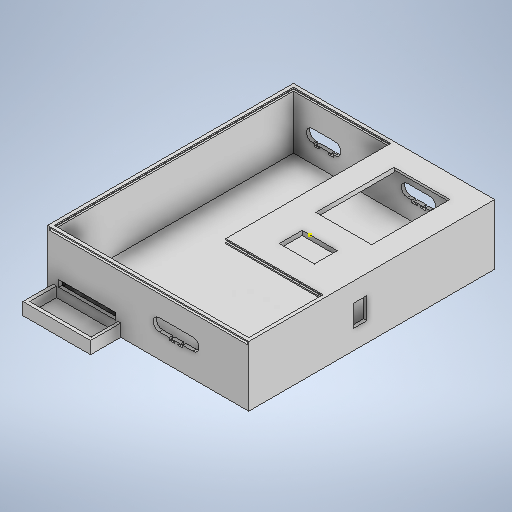
# Autodesk Inventor part: Main Case
Saved by Autodesk Inventor 2025.3 (Build 293356000, 356)
## iProperties
Created: 2026-02-11
Part Number: Main Case
Material: Generic
Document SubType Name: Modeling
Designer: Maulana
Density: 1 g/cm^3
Appearance: Default
Mass: 297.641 g
Surface Area: 2038.3 cm^2
Volume: 297.641 cm^3
Author: Maulana
Autodesk Inventor part; units mm, degrees
sketch "Sketch1" plane through (0, 0, 0) normal (0, 1, 0) x (-1, 0, 0)
  line L0 (-122, 107) -> (122, 107)
  line L1 (122, 107) -> (122, -107)
  line L2 (122, -107) -> (-122, -107)
  line L3 (-122, -107) -> (-122, 107)
  line L4 (-122, 107) -> (122, -107) construction
  line L5 (122, 107) -> (-122, -107) construction
  line L6 (-125, 110) -> (125, 110)
  line L7 (125, 110) -> (125, -110)
  line L8 (125, -110) -> (-125, -110)
  line L9 (-125, -110) -> (-125, 110)
  line L10 (-125, 110) -> (125, -110) construction
  line L11 (125, 110) -> (-125, -110) construction
  line L12 (122, 107) -> (-52, 107)
  line L13 (-52, 107) -> (-52, -107)
  line L14 (125, 110) -> (-55, 110)
  line L15 (-55, 110) -> (-55, -110)
  point P0 (0, 0)
  dimension "d0" = 244
  dimension "d1" = 214
  dimension "d2" = 250
  dimension "d3" = 220
  dimension "d111" = 174
  dimension "d112" = 180
  constraints: 32 end point, 4 midpoint, 4 parallel, 4 perpendicular, 4 point on line, 2 horizontal
  measures "d0" distance of L1.end L2.end
  measures "d1" distance of L0.end L1.end
  measures "d2" distance of L7.end L8.end
  measures "d3" distance of L6.end L7.end
  measures "d111" distance of L0.end L12.end
  measures "d112" distance of L6.end L14.end
extrude "Extrusion1" add sketch "Sketch1" along normal blind 54 contours L0 L15 L6 L7 L8 L2 L1 | L13 L2 L15 L0
sketch "Sketch2" plane through (0, 0, 0) normal (0, -1, 0) x (1, 0, 0)
  line L0 (123.5, 110) -> (-123.5, 110)
  line L1 (-123.5, 110) -> (-123.5, -110)
  line L2 (-123.5, -110) -> (123.5, -110)
  line L3 (123.5, -110) -> (123.5, 110)
  line L4 (123.5, 110) -> (-123.5, -110) construction
  line L5 (-123.5, 110) -> (123.5, -110) construction
  line L6 (55, 110) -> (55, -110) projected
  line L7 (55, 110) -> (55, -110)
  point P0 (0, 0)
  dimension "d6" = 247
  dimension "d7" = 220
  constraints: 14 end point, 2 midpoint, 2 parallel, 2 perpendicular, 1 horizontal
  measures "d6" distance of L2.end L1.end
  measures "d7" distance of L1.end L0.end
extrude "Extrusion2" add sketch "Sketch2" against normal blind 3 contours L6 L2 L1 L0
sketch "Sketch3" plane through (-125, 0, 110) normal (0, 0, 1) x (1, 0, 0)
  line L0 (0, 0) -> (0, 54) projected
  line L1 (0, 27) -> (100, 27)
  circle A0 centre (100, 27) radius 8
  circle A1 centre (100, 27) radius 5.5
  line L2 (100, 35) -> (115, 35)
  line L3 (115, 35) -> (115, 19)
  line L4 (115, 19) -> (100, 19)
  line L5 (100, 19) -> (100, 35)
  line L6 (100, 32.5) -> (115, 32.5)
  line L7 (115, 32.5) -> (115, 21.5)
  line L8 (115, 21.5) -> (100, 21.5)
  line L9 (100, 21.5) -> (100, 32.5)
  line L10 (100, 32.5) -> (109, 32.5)
  line L11 (109, 32.5) -> (109, 34.5)
  line L12 (109, 34.5) -> (113.5, 34.5)
  line L13 (113.5, 34.5) -> (113.5, 33.5)
  line L14 (113.5, 33.5) -> (111, 33.5)
  line L15 (111, 33.5) -> (111, 32.5)
  line L16 (100, 27) -> (115, 27)
  line L17 (109, 21.5) -> (109, 19.5)
  line L18 (109, 19.5) -> (113.5, 19.5)
  line L19 (113.5, 19.5) -> (113.5, 20.5)
  line L20 (113.5, 20.5) -> (111, 20.5)
  line L21 (111, 20.5) -> (111, 21.5)
  point P0 (125, 0)
  dimension "d10" = 100
  dimension "d11" = 16
  dimension "d12" = 11
  dimension "d13" = 15
  dimension "d14" = 9
  dimension "d15" = 2
  dimension "d16" = 4.5
  dimension "d17" = 2.5
  constraints: 42 end point, 6 symmetric about line, 5 parallel, 5 perpendicular, 4 point on circle, 4 point on line, 3 horizontal, 2 centre point, 2 coincident, 2 midpoint, 1 vertical
  measures "d10" distance of L1.start L1.end
  measures "d11" diameter of A0
  measures "d12" diameter of A1
  measures "d13" distance of L3.end L4.end
  measures "d14" distance of L6.start L10.end
  measures "d15" distance of L10.end L11.end
  measures "d16" distance of L11.end L12.end
  measures "d17" distance of L13.end L14.end
extrude "Extrusion3" cut sketch "Sketch3" against normal blind 38 contours A1 L5 L1 | L1 L5 A1 | L16 A1 L5 | L5 A1 L16 | L6 A0 L16 A1 | A1 L16 A0 L8 | L6 L3 L16 A0 | A0 L16 L3 L8 | L8 L21 L20 L19 L18 L17
ref_plane "Work Plane2" through (-10, 21.5, 110) normal (-1, 0, 0) x (0, 0, 1)
mirror "Mirror1" about plane through (-10, 21.5, 110) normal (-1, 0, 0) of "Extrusion3"
sketch "Sketch5" plane through (125, 0, -110) normal (0, 0, -1) x (-1, 0, 0)
  line L0 (250, 6) -> (250, 25)
  line L1 (250, 25) -> (230, 25)
  circle A0 centre (230, 25) radius 8
  circle A1 centre (230, 25) radius 5.5
  line L2 (230, 33) -> (220, 33)
  line L3 (220, 33) -> (220, 17)
  line L4 (220, 17) -> (230, 17)
  line L5 (230, 17) -> (230, 33)
  line L6 (230, 30.5) -> (220, 30.5)
  line L7 (220, 30.5) -> (220, 19.5)
  line L8 (220, 19.5) -> (230, 19.5)
  line L9 (230, 19.5) -> (230, 30.5)
  line L10 (230, 30.5) -> (228.5, 30.5)
  line L11 (228.5, 30.5) -> (228.5, 32.5)
  line L12 (228.5, 32.5) -> (224, 32.5)
  line L13 (224, 32.5) -> (224, 31.5)
  line L14 (224, 31.5) -> (226.5, 31.5)
  line L15 (226.5, 31.5) -> (226.5, 30.5)
  line L16 (230, 25) -> (230, 0)
  line L17 (70, 0) -> (250, 0) projected
  line L18 (250, 0) -> (230, 0)
  line L19 (250, 0) -> (230, 0)
  line L20 (228.5, 19.5) -> (228.5, 17.5)
  line L21 (228.5, 17.5) -> (224, 17.5)
  line L22 (224, 17.5) -> (224, 18.5)
  line L23 (224, 18.5) -> (226.5, 18.5)
  line L24 (226.5, 18.5) -> (226.5, 19.5)
  point P0 (125, 0)
  point P1 (121.8464, -1.1281)
  point P2 (220.8464, 22.8719)
  point P3 (228.3464, 12.8719)
  point P4 (227.2161, 32.5)
  point P5 (225.3363, 31.5)
  point P6 (0, 0)
  point P7 (1.5, 0)
  dimension "d36" = 20
  dimension "d37" = 16
  dimension "d38" = 11
  dimension "d39" = 10
  dimension "d40" = 1.5
  dimension "d41" = 2
  dimension "d42" = 4.5
  dimension "d43" = 2.5
  dimension "d44" = 1
  dimension "d45" = 1
  dimension "d63" = 25
  dimension "d103" = 19
  dimension "d106" = 20
  constraints: 48 end point, 8 perpendicular, 6 point on line, 6 symmetric about line, 4 parallel, 4 point on circle, 3 horizontal, 2 centre point, 2 coincident, 2 collinear
  measures "d36" distance of L0.end L1.end
  measures "d37" diameter of A0
  measures "d38" diameter of A1
  measures "d39" distance of L4.end L3.end
  measures "d40" distance of L6.start L10.end
  measures "d41" distance of L10.end L11.end
  measures "d42" distance of L11.end L12.end
  measures "d43" distance of L13.end L14.end
  measures "d44" distance of L14.end L15.end
  measures "d45" distance of L12.end L13.end
  measures "d63" distance of L16.start L16.end
  measures "d103" distance of L0.start L0.end
  measures "d106" distance of L17.end L16.end
extrude "Extrusion5" cut sketch "Sketch5" against normal blind 10 contours A1 L5 L1 | L1 L5 A1 | L5 A1 | A1 L8 A0 L6 | L21 L22 L23 A0 | A0 L23 L24 L8 L20 L21 | L6 A0 L8 L3
ref_plane "Work Plane4" through (-95, 19.5, -110) normal (-1, 0, 0) x (0, 0, 1)
mirror "Mirror3" about plane through (-95, 19.5, -110) normal (-1, 0, 0) of "Extrusion5"
sketch "Sketch6" plane through (125, 0, -110) normal (0, 0, -1) x (-1, 0, 0)
  circle A0 centre (125, 25) radius 8
  circle A1 centre (125, 25) radius 5.5
  line L0 (125, 33) -> (135, 33)
  line L1 (135, 33) -> (135, 17)
  line L2 (135, 17) -> (125, 17)
  line L3 (125, 30.5) -> (135, 30.5)
  line L4 (135, 19.5) -> (125, 19.5)
  line L5 (125, 30.5) -> (129, 30.5)
  line L6 (129, 30.5) -> (129, 32.5)
  line L7 (129, 32.5) -> (133.5, 32.5)
  line L8 (133.5, 25) -> (133.5, 24.983)
  line L9 (133.5, 31.5) -> (131, 31.5)
  line L10 (131, 31.5) -> (131, 30.5)
  line L11 (116.2614, 18.9998) -> (135.2614, 18.9998) construction
  line L12 (133.5, 32.5) -> (133.5, 31.5)
  line L13 (250, 0) -> (250, 54) projected
  line L14 (250, 0) -> (125, 0)
  line L15 (70, 0) -> (250, 0) projected
  line L16 (125, 25) -> (125, 0)
  line L17 (125, 33) -> (125, 25)
  line L18 (125, 30.5) -> (125, 33)
  line L19 (131, 30.5) -> (131, 31.5)
  line L20 (135, 33) -> (135, 17)
  line L21 (125, 17) -> (135, 17)
  line L22 (125, 25) -> (135, 25)
  line L23 (129, 19.5) -> (129, 17.5)
  line L24 (129, 17.5) -> (133.5, 17.5)
  line L25 (133.5, 18.5) -> (131, 18.5)
  line L26 (131, 18.5) -> (131, 19.5)
  line L27 (133.5, 17.5) -> (133.5, 18.5)
  point P0 (125, 0)
  point P1 (219.2081, 3.6104)
  point P2 (112.7081, 17.6104)
  point P3 (127.7081, 27.6104)
  point P4 (0, 0)
  point P5 (1.5, 0)
  dimension "d50" = 16
  dimension "d51" = 11
  dimension "d54" = 2
  dimension "d55" = 4.5
  dimension "d56" = 2.5
  dimension "d57" = 1.5
  dimension "d104" = 25
  dimension "d105" = 125
  constraints: 52 end point, 6 perpendicular, 6 symmetric about line, 5 point on line, 4 collinear, 4 horizontal, 3 parallel, 2 point on circle, 2 vertical, 1 centre point, 1 coincident, 1 midpoint, 1 vertical alignment, 2 other
  measures "d51" diameter of A1
  measures "d54" distance of L5.end L6.end
  measures "d55" distance of L6.end L7.end
  measures "d56" distance of L9.start L9.end
  measures "d57" distance between parallel lines of L1 L8
  measures "d104" distance of L16.start L14.end
  measures "d105" distance of L13.start L14.end
extrude "Extrusion6" cut sketch "Sketch6" against normal blind 10 contours L3 A0 L22 A1 | L17 L16 A1 | A1 L22 L17 | L23 L4 A0 | A0 L4 L26 L25 L27 L24 L23 | L16 L22 A1 | A1 L22 A0 L4 | L3 L1 L22 A0 | A0 L22 L1 L4
ref_plane "Work Plane5" through (-10, 19.5, -110) normal (1, 0, 0) x (0, 0, -1)
mirror "Mirror4" about plane through (-10, 19.5, -110) normal (1, 0, 0) of "Extrusion6"
sketch "Sketch7" plane through (122, 50, 107) normal (0, 0, -1) x (-1, 0, 0)
  line L0 (70, -47) -> (244, -47) projected
  line L1 (75.0855, -47) -> (75.0855, -50)
  line L2 (75.0855, -50) -> (75.0855, -47)
  line L3 (0, -47) -> (184, -47)
  line L4 (184, -47) -> (184, -39)
  line L5 (184, -39) -> (239, -39)
  line L6 (239, -39) -> (239, -47)
  line L7 (184, -39) -> (194, -39)
  line L8 (239, -39) -> (229, -39)
  line L9 (194, -34.8824) -> (194, -33)
  line L10 (194, -33) -> (229, -33)
  line L11 (229, -33) -> (229, -34.8824)
  line L12 (244, -47) -> (244, 4) projected
  line L13 (184, -47) -> (211.5, -47)
  line L14 (211.5, -47) -> (211.5, -39)
  line L15 (237, -39) -> (237, -33)
  line L16 (237, -33) -> (186, -33)
  line L17 (186, -33) -> (186, -39)
  line L18 (186, -45) -> (237, -33) construction
  line L19 (237, -45) -> (186, -33) construction
  line L20 (186, -39) -> (237, -39)
  point P0 (122, -50)
  point P1 (244, 4)
  point P2 (239, -43)
  point P3 (2, -35)
  point P4 (245, -35)
  point P5 (247, -38)
  point P6 (186, -39)
  point P7 (237, -39)
  dimension "d65" = 8
  dimension "d66" = 55
  dimension "d67" = 10
  dimension "d68" = 10
  dimension "d69" = 6
  dimension "d89" = 5
  dimension "d90" = 51
  constraints: 38 end point, 7 point on line, 4 midpoint, 3 perpendicular, 3 vertical, 2 collinear, 1 horizontal, 1 parallel, 6 other
  measures "d65" distance of L3.end L4.end
  measures "d66" distance of L4.end L5.end
  measures "d67" distance of L4.end L7.end
  measures "d68" distance of L5.end L8.end
  measures "d69" distance of L7.end L9.end
  measures "d90" distance of L18.start L19.start
extrude "Extrusion7" cut sketch "Sketch7" against normal blind 10 contours L5 L17 L16 L10 L15
sketch "Sketch17" plane through (-125, 0, 110) normal (0, 0, 1) x (1, 0, 0)
  line L0 (10, 11) -> (61, 11) projected
  line L1 (35.5, 11) -> (35.5, 0)
  line L2 (177, 3) -> (3, 3) projected
  line L3 (35.5, -2) -> (63, -2)
  line L4 (63, -2) -> (63, 2)
  line L5 (63, 2) -> (8, 2)
  line L6 (8, 2) -> (8, -2)
  line L7 (8, -2) -> (63, 2) construction
  line L8 (63, -2) -> (8, 2) construction
  line L9 (180, 0) -> (0, 0) projected
  line L10 (8, 0) -> (63, 0)
  point P0 (125, 0)
  point P1 (247, 3)
  point P2 (250, 0)
  point P3 (248.5, 0)
  dimension "d91" = 55
  dimension "d92" = 4
  constraints: 16 end point, 5 midpoint, 3 point on line, 2 parallel, 2 perpendicular, 1 horizontal
  measures "d91" distance of L6.end L3.end
  measures "d92" distance of L3.end L4.end
extrude "Extrusion11" add sketch "Sketch17" along normal blind 24
sketch "Sketch18" plane through (-117, 2, 110) normal (0, 1, 0) x (1, 0, 0)
  line L0 (0, 0) -> (0, -24) projected
  line L1 (0, 0) -> (55, 0)
  line L2 (55, 0) -> (55, -24)
  line L3 (55, -24) -> (0, -24)
  line L4 (0, -24) -> (0, 0)
  line L5 (0, 0) -> (-3, 0)
  line L6 (55, 0) -> (58, 0)
  line L7 (-3, 0) -> (57.4885, 0)
  line L8 (57.4885, 0) -> (57.4885, -27)
  line L9 (57.4885, -27) -> (-3, -27)
  line L10 (-3, -27) -> (-3, 0)
  point P0 (117, 110)
  point P1 (57.4885, 0)
  dimension "d95" = 3
  dimension "d96" = 3
  dimension "d97" = 27
  constraints: 20 end point, 4 horizontal, 4 parallel, 2 perpendicular
  measures "d95" distance of L0.start L5.end
  measures "d96" distance of L1.end L6.end
  measures "d97" distance of L7.end L8.end
extrude "Extrusion12" add sketch "Sketch18" along normal blind 9 and the other way blind 2 contours L0 L3 L2 L6 L8 L9 L10 L5
sketch "Sketch20" plane through (0, 54, 0) normal (0, 1, 0) x (1, 0, 0)
  point P0 (0, 0)
sketch "Sketch21" plane through (0, 54, 0) normal (0, 1, 0) x (1, 0, 0)
  line L0 (55, 110) -> (-125, 110) projected
  line L1 (55, 110) -> (-35, 110)
  line L2 (-35, 110) -> (-35, -40.5)
  line L3 (-35, -40.5) -> (55, -40.5)
  line L4 (55, -40.5) -> (55, 110)
  point P0 (0, 0)
  dimension "d113" = 90
  dimension "d114" = 150.5
  constraints: 8 end point, 2 parallel, 1 horizontal, 1 perpendicular
  measures "d113" distance of L3.end L2.end
  measures "d114" distance of L2.end L1.end
extrude "Extrusion14" add sketch "Sketch21" against normal blind 4
sketch "Sketch22" plane through (0, 54, 0) normal (0, 1, 0) x (1, 0, 0)
  line L0 (55, 110) -> (-125, 110) projected
  line L1 (-35, 110) -> (10, 110)
  line L2 (10, 110) -> (10, -40.5)
  line L3 (52, -40.5) -> (-35, -40.5) projected
  line L4 (10, 110) -> (10, 90)
  line L5 (-35, -40.5) -> (-35, 107) projected
  line L6 (-35, 90) -> (-15, 90)
  line L7 (-35, 90) -> (-15, 90) construction
  line L8 (55, -110) -> (55, 110) projected
  line L9 (55, 90) -> (35, 90)
  line L10 (55, 90) -> (75, 90) construction
  line L11 (-15, 90) -> (35, 90)
  line L12 (35, 90) -> (35, 20)
  line L13 (35, 20) -> (-15, 20)
  line L14 (-15, 20) -> (-15, 90)
  point P0 (0, 0)
  dimension "d117" = 45
  dimension "d118" = 20
  dimension "d119" = 20
  dimension "d120" = 0
  dimension "d121" = 20
  dimension "d122" = 180
  dimension "d123" = 70
  constraints: 22 end point, 5 point on line, 4 perpendicular, 3 horizontal, 2 collinear, 2 parallel, 1 midpoint
  measures "d117" distance of L1.start L1.end
  measures "d118" distance of L1.end L4.end
  measures "d119" distance of L6.start L6.end
  measures "d120" distance between parallel lines of L6 L7
  measures "d121" distance of L9.start L9.end
  measures "d122" angle of L9 L10
  measures "d123" distance of L11.end L12.end
extrude "Extrusion15" cut sketch "Sketch22" against normal blind 4 contours L11 L12 L13 L2 | L2 L13 L14 L11
sketch "Sketch23" plane through (0, 54, 0) normal (0, 1, 0) x (1, 0, 0)
  line L0 (52, -40.5) -> (-35, -40.5) projected
  line L1 (8.5, -40.5) -> (8.5, 20)
  line L2 (-15, 20) -> (35, 20) projected
  line L3 (-35, -40.5) -> (-35, 107) projected
  line L4 (-35, -10.25) -> (55, -10.25)
  line L5 (-35, -10.25) -> (55, -10.25) construction
  line L6 (24.25, -20.5) -> (-7.25, -20.5)
  line L7 (-7.25, -20.5) -> (-7.25, 0)
  line L8 (-7.25, 0) -> (24.25, 0)
  line L9 (24.25, 0) -> (24.25, -20.5)
  line L10 (24.25, -20.5) -> (-7.25, 0) construction
  line L11 (-7.25, -20.5) -> (24.25, 0) construction
  point P0 (0, 0)
  point P1 (8.5, -10.25)
  dimension "d126" = 90
  dimension "d127" = 0
  dimension "d128" = 31.5
  constraints: 18 end point, 4 midpoint, 3 point on line, 2 horizontal, 2 parallel, 2 perpendicular, 1 collinear, 1 vertical
  measures "d126" distance of L4.start L4.end
  measures "d127" distance between parallel lines of L4 L5
  measures "d128" distance of L7.end L8.end
extrude "Extrusion16" cut sketch "Sketch23" against normal blind 4 contours L6 L7 L4 L1 | L1 L4 L9 L6 | L4 L7 L8 L1 | L1 L8 L9 L4
sketch "Sketch24" plane through (55, 0, 110) normal (1, 0, 0) x (0, 0, -1)
  line L0 (99.75, 54.0966) -> (99.75, 0)
  line L1 (217, 3) -> (3, 3) projected
  line L2 (0, 0) -> (0, 54) projected
  line L3 (0, 27) -> (220, 27)
  line L4 (220, 0) -> (220, 54) projected
  line L5 (93.75, 17.25) -> (105.75, 17.25)
  line L6 (105.75, 17.25) -> (105.75, 36.75)
  line L7 (105.75, 36.75) -> (93.75, 36.75)
  line L8 (93.75, 36.75) -> (93.75, 17.25)
  line L9 (93.75, 17.25) -> (105.75, 36.75) construction
  line L10 (105.75, 17.25) -> (93.75, 36.75) construction
  point P0 (110, 0)
  point P1 (99.75, 27)
  dimension "d131" = 12
  dimension "d132" = 19.5
  constraints: 16 end point, 4 midpoint, 2 parallel, 2 perpendicular, 2 point on line, 1 horizontal
  measures "d131" distance of L7.end L6.end
  measures "d132" distance of L6.end L5.end
extrude "Extrusion17" cut sketch "Sketch24" against normal blind 4
sketch "Sketch27" plane through (-35, 54, -107) normal (-1, 0, 0) x (0, 0, 1)
  line L0 (17, 0) -> (17, -4) projected
  line L1 (17, -4) -> (7, -4)
  line L2 (147.5, -4) -> (0, -4) projected
  line L3 (7, -4) -> (17, -4)
  line L4 (17, -4) -> (17, -2)
  line L5 (17, -2) -> (7, -2)
  line L6 (7, -2) -> (7, -4)
  point P0 (107, -54)
  dimension "d135" = 10
  constraints: 10 end point, 2 parallel, 1 horizontal, 1 midpoint, 1 perpendicular, 1 point on line
  measures "d135" distance of L0.end L1.end
extrude "Extrusion18" cut sketch "Sketch27" against normal blind 70
sketch "Sketch29" plane through (-125, 54, 110) normal (0, 0, 1) x (1, 0, 0)
  line L0 (3, -51) -> (3, 0) projected
  line L1 (3, 0) -> (3, -1)
  line L2 (3, -1) -> (1.5, -1)
  line L3 (1.5, -1) -> (1.5, -3)
  line L4 (1.5, -3) -> (3, -3)
  line L5 (1.5, -1) -> (178.5, -1)
  line L6 (178.5, -1) -> (178.5, -3)
  line L7 (178.5, -3) -> (1.5, -3)
  line L8 (1.5, -3) -> (1.5, -1)
  line L9 (90, -4) -> (90, 0) projected
  line L10 (90, -1) -> (90, -3)
  line L11 (90, -1) -> (91.5, -1)
  line L12 (91.5, -1) -> (91.5, -3)
  line L13 (90, -3) -> (91.5, -3)
  point P0 (125, -54)
  point P1 (3, -1)
  dimension "d140" = 1
  dimension "d141" = 1.5
  dimension "d142" = 2
  dimension "d143" = 177
  dimension "d144" = 2
  dimension "d147" = 1.5
  constraints: 24 end point, 6 point on line, 4 perpendicular, 2 horizontal, 2 midpoint, 2 parallel, 1 collinear
  measures "d140" distance of L0.end L1.end
  measures "d141" distance of L1.end L2.end
  measures "d142" distance of L2.end L3.end
  measures "d143" distance of L6.end L7.end
  measures "d144" distance of L5.end L6.end
  measures "d147" distance of L10.start L11.end
extrude "Extrusion20" cut sketch "Sketch29" against normal blind 218.5 contours L4 L3 L2 L0 | L0 L5 L9 L7 | L9 L5 L12 L7
sketch "Sketch30" plane through (-125, 54, 110) normal (0, 0, 1) x (1, 0, 0)
  line L0 (91.5, -1) -> (178.5, -1)
  line L1 (178.5, -1) -> (178.5, -3)
  line L2 (178.5, -3) -> (91.5, -3)
  line L3 (91.5, -3) -> (91.5, -1)
  point P0 (125, -54)
  dimension "d148" = 87
  dimension "d149" = 2
  constraints: 8 end point, 2 parallel, 1 horizontal, 1 perpendicular
  measures "d148" distance of L1.end L2.end
  measures "d149" distance of L0.end L1.end
extrude "Extrusion21" cut sketch "Sketch30" against normal blind 71
body "Solid1"
